Autodesk Fusion 360 part; units mm, degrees
(part 2 of 2)
  line L234 (5.7078, -72.7576) -> (5.7078, -72.8052)
  arc A116 (5.4973, -73.1059) -> (5.7078, -72.8052) centre (5.3878, -72.8052) ccw
  line L235 (5.4973, -73.1059) -> (4.0203, -73.6434)
  line L236 (4.0203, -73.6434) -> (4.0203, -74.2756)
  line L237 (4.0203, -74.2756) -> (5.4973, -74.8131)
  arc A117 (5.7078, -75.1138) -> (5.4973, -74.8131) centre (5.3878, -75.1138) ccw
  line L238 (5.7078, -75.1138) -> (5.7078, -75.1614)
  arc A118 (5.4973, -75.4621) -> (5.7078, -75.1614) centre (5.3878, -75.1614) ccw
  line L239 (5.4973, -75.4621) -> (4.0203, -75.9996)
  line L240 (4.0203, -75.9996) -> (4.0203, -76.6318)
  line L241 (4.0203, -76.6318) -> (5.4973, -77.1693)
  arc A119 (5.7078, -77.47) -> (5.4973, -77.1693) centre (5.3878, -77.47) ccw
  line L242 (5.7078, -77.47) -> (5.7078, -77.5176)
  arc A120 (5.4973, -77.8183) -> (5.7078, -77.5176) centre (5.3878, -77.5176) ccw
  line L243 (5.4973, -77.8183) -> (4.0203, -78.3558)
  line L244 (4.0203, -78.3558) -> (4.0203, -78.988)
  line L245 (4.0203, -78.988) -> (5.4973, -79.5255)
  arc A121 (5.7078, -79.8262) -> (5.4973, -79.5255) centre (5.3878, -79.8262) ccw
  line L246 (5.7078, -79.8262) -> (5.7078, -79.8737)
  arc A122 (5.4973, -80.1745) -> (5.7078, -79.8737) centre (5.3878, -79.8737) ccw
  line L247 (5.4973, -80.1745) -> (4.0203, -80.712)
  line L248 (4.0203, -80.712) -> (4.0203, -81.3442)
  line L249 (4.0203, -81.3442) -> (5.4973, -81.8817)
  arc A123 (5.7078, -82.1824) -> (5.4973, -81.8817) centre (5.3878, -82.1824) ccw
  line L250 (5.7078, -82.1824) -> (5.7078, -82.2299)
  arc A124 (5.4973, -82.5306) -> (5.7078, -82.2299) centre (5.3878, -82.2299) ccw
  line L251 (5.4973, -82.5306) -> (4.0203, -83.0682)
  line L252 (4.0203, -83.0682) -> (4.0203, -83.7004)
  line L253 (4.0203, -83.7004) -> (5.4973, -84.2379)
  arc A125 (5.7078, -84.5386) -> (5.4973, -84.2379) centre (5.3878, -84.5386) ccw
  line L254 (5.7078, -84.5386) -> (5.7078, -84.5861)
  arc A126 (5.4973, -84.8868) -> (5.7078, -84.5861) centre (5.3878, -84.5861) ccw
  line L255 (5.4973, -84.8868) -> (4.0203, -85.4244)
  line L256 (4.0203, -85.4244) -> (4.0203, -86.0565)
  line L257 (4.0203, -86.0565) -> (5.4973, -86.5941)
  arc A127 (5.707, -86.9185) -> (5.4973, -86.5941) centre (5.3878, -86.8948) ccw
  line L258 (25.7073, -80.4187) -> (25.7073, -78.3187) construction
  line L259 (5.707, -80.4185) -> (25.7073, -80.4185)
  line L260 (25.7073, -80.4185) -> (25.7073, -78.3187)
  line L261 (25.7073, -78.3187) -> (5.707, -78.3187)
  line L262 (5.707, -78.3187) -> (5.707, -80.4185)
  dimension "d15" = 2.1
  constraint coincident L1 L258.start
  constraint horizontal L259
  constraint vertical L260
  constraint horizontal L261
  constraint vertical L262
  measures "d15" distance of L258.start L258.end
extrude "Extrude3" add sketch "Sketch4" along normal blind 10.5 contours L1 L246 L259 L260 L261 L262 bodies 2
extrude "Extrude4" cut sketch "Sketch1 (2)" against normal blind 20 contours L19 L20 A0 | L19 L20 A0 | L19 L20 A0 | L19 L20 A0 bodies 2
extrude "Extrude3'" add sketch "Sketch4" against normal blind 35.5 contours L1 L246 L259 L260 L261 L262 sketch seen with x (0, -1, 0) y (0, 0, 1) z (-1, 0, 0) at (-11.5203, 12.5, -24.0203) bodies 1 in component "Rack Gear (64 teeth)"
extrude "Extrude4'" cut sketch "Sketch1 (2)" against normal blind 25 contours A1 sketch seen with x (0, -1, 0) y (0, 0, 1) z (-1, 0, 0) at (-11.5203, 12.5, -24.0203) bodies 1 in component "Rack Gear (64 teeth)"
extrude "Extrude5" cut sketch "Sketch1 (2)" against normal blind 155 contours L3 L8 L9 L23 L25 L28 | L8 L9 L27 L28 | L3 L8 L9 L24 L26 L29 | L8 L9 L27 L29 sketch seen with x (0, -1, 0) y (0, 0, 1) z (-1, 0, 0) at (-11.5203, 12.5, -24.0203) bodies 1 in component "Rack Gear (64 teeth)"
extrude "Extrude6" add sketch "Sketch1 (2)" against normal blind 1.6 contours L3 L8 L9 L23 L25 L28 | L8 L9 L27 L28 | L3 L8 L9 L24 L26 L29 | L8 L9 L27 L29 sketch seen with x (0, -1, 0) y (0, 0, 1) z (-1, 0, 0) at (-11.5203, 12.5, -24.0203) bodies 1 in component "Rack Gear (64 teeth)"
extrude "Extrude7" add sketch "Sketch3" along normal blind 5 contours L4 L5 L6 L7 L8 L9 sketch seen with x (0, -1, 0) y (0, 0, 1) z (-1, 0, 0) at (-11.5203, 12.5, -24.0203) bodies 1 in component "Rack Gear (64 teeth)"
extrude "Extrude5'" add sketch "Sketch2 (2)" along normal blind 5 contours L4 L5 L6 L7 L8 L9 bodies 2
component "Rack Gear (64 teeth)" placed x (0, 0, -1) y (-1, 0, 0) z (0, 1, 0) at (12.5, 24.0203, -11.5203)
